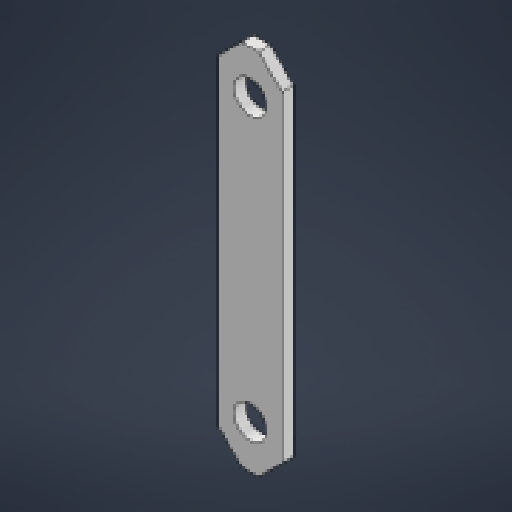
# Autodesk Inventor part: Endgame brake pad polycarb
Saved by Autodesk Inventor 2023.2 (Build 272271030, 271C)
## iProperties
Created: 2023-04-07
Part Number: Endgame brake pad polycarb
Material: Generic
Document SubType Name: Modeling
Designer: Main Account
Density: 1 g/cm^3
Appearance: Default
Author: Main Account
Autodesk Inventor part; units mm, degrees
ref_plane "YZ Plane" through (0, 0, 0) normal (1, 0, 0) x (0, 1, 0)
ref_plane "XZ Plane" through (0, 0, 0) normal (0, 1, 0) x (-1, 0, 0)
ref_plane "XY Plane" through (0, 0, 0) normal (0, 0, 1) x (1, 0, 0)
sketch "Sketch1" plane through (0, 0, 0) normal (0, 0, 1) x (1, 0, 0)
  circle A0 centre (-1.1684, -19.05) radius 2.1844 projected
  circle A1 centre (-1.1684, 19.05) radius 2.1844 projected
  line L0 (3.9688, -24.2345) -> (3.9688, 38.1) construction
  line L1 (-0.0172, -24.9245) -> (-2.3196, -24.9245)
  line L2 (-5.4946, -21.7495) -> (-5.4946, 21.7495)
  line L3 (-2.3196, 24.9245) -> (-0.0172, 24.9245)
  line L4 (3.1578, 21.7495) -> (3.1578, -21.7495)
  line L5 (-2.3196, -24.9245) -> (-5.4946, -21.7495)
  line L6 (-0.0172, -24.9245) -> (3.1578, -21.7495)
  line L7 (-0.0172, 24.9245) -> (3.1578, 21.7495)
  line L8 (-5.4946, 21.7495) -> (-2.3196, 24.9245)
  point P0 (0, 0)
  point P1 (3.1578, -24.9245)
  point P2 (-5.4946, 24.9245)
  point P3 (-5.4946, -24.9245)
  point P4 (3.1578, 24.9245)
  dimension "d0" = 3.175
  dimension "d1" = 3.175
  dimension "d2" = 3.175
  dimension "d3" = 3.175
  dimension "d4" = 3.175
  dimension "d5" = 3.175
  dimension "d6" = 3.175
  dimension "d7" = 3.175
  constraints: 16 end point, 8 point on line, 2 parallel, 1 horizontal, 1 perpendicular
  measures "d0" distance of L1.end point (-5.495, -24.925)
  measures "d1" distance of L2.start point (-5.495, -24.925)
  measures "d2" distance of L1.start point (3.158, -24.925)
  measures "d3" distance of L4.end point (3.158, -24.925)
  measures "d4" distance of L3.end point (3.158, 24.925)
  measures "d5" distance of L4.start point (3.158, 24.925)
  measures "d6" distance of L2.end point (-5.495, 24.925)
  measures "d7" distance of L3.start point (-5.495, 24.925)
extrude "Extrusion1" add sketch "Sketch1" along normal blind 1.5875
equation "\"d1\" = d0"
equation "\"d2\" = d0"
equation "\"d3\" = d2"
equation "\"d4\" = d0"
equation "\"d5\" = d4"
equation "\"d6\" = d0"
equation "\"d7\" = d6"
body "Solid1"
